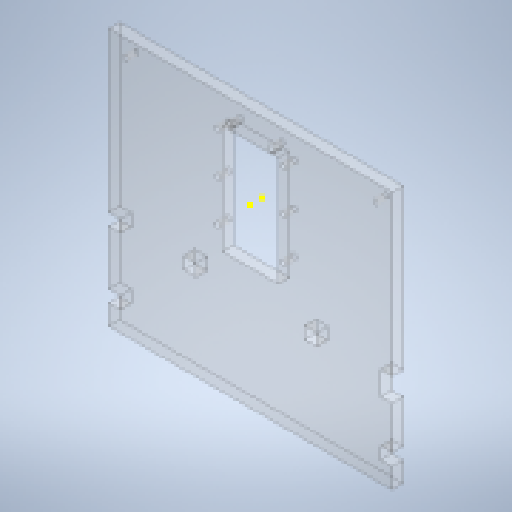
# Autodesk Inventor part: real_waist
Saved by Autodesk Inventor 2024 (Build 280153000, 153)
## iProperties
Created: 2024-09-06
Part Number: real_waist
Material: PMMA 플라스틱
Document SubType Name: Modeling
Designer: Eungang
Density: 1.188 g/cm^3
Appearance: 폴리카보네이트 - 선명
Mass: 126.494 g
Surface Area: 420.568 cm^2
Volume: 106.476 cm^3
Author: Eungang
Autodesk Inventor part; units mm, degrees
ref_plane "YZ Plane" through (0, 0, 0) normal (1, 0, 0) x (0, 1, 0)
ref_plane "XZ Plane" through (0, 0, 0) normal (0, 1, 0) x (-1, 0, 0)
ref_plane "XY Plane" through (0, 0, 0) normal (0, 0, 1) x (1, 0, 0)
sketch "스케치1" plane through (0, 0, 0) normal (0, 0, 1) x (1, 0, 0)
  arc A0 (-19.5808, 6.2636) -> (-20.1, 4.5766) centre (-17.1, 4.5766) ccw projected
  line L0 (-20.1, -39.6766) -> (-20.1, 4.5766) projected
  arc A1 (-20.1, -39.6766) -> (-19.5808, -41.3636) centre (-17.1, -39.6766) ccw projected
  line L1 (-15.8929, -46.7869) -> (-19.5808, -41.3636) projected
  arc A2 (-15.8929, -46.7869) -> (-13.4121, -48.1) centre (-13.4121, -45.1) ccw projected
  line L2 (13.4121, -48.1) -> (-13.4121, -48.1) projected
  arc A3 (13.4121, -48.1) -> (15.8929, -46.7869) centre (13.4121, -45.1) ccw projected
  line L3 (19.5808, -41.3636) -> (15.8929, -46.7869) projected
  arc A4 (19.5808, -41.3636) -> (20.1, -39.6766) centre (17.1, -39.6766) ccw projected
  line L4 (20.1, 4.5766) -> (20.1, -39.6766) projected
  arc A5 (20.1, 4.5766) -> (19.5808, 6.2636) centre (17.1, 4.5766) ccw projected
  line L5 (15.5953, 12.1246) -> (19.5808, 6.2636) projected
  arc A6 (15.5953, 12.1246) -> (13.9414, 13) centre (13.9414, 11) ccw projected
  line L6 (7.65, 13) -> (13.9414, 13) projected
  arc A7 (9.15, 11.5) -> (7.65, 13) centre (7.65, 11.5) ccw projected
  line L7 (9.15, 11.5) -> (9.15, 10) projected
  arc A8 (9.15, 10) -> (11.5, 7.65) centre (11.5, 10) ccw projected
  line L8 (11.5, 7.65) -> (13.5, 7.65) projected
  arc A9 (14.5, 6.65) -> (13.5, 7.65) centre (13.5, 6.65) ccw projected
  line L9 (14.5, 6.65) -> (14.5, -36.15) projected
  arc A10 (13.5, -37.15) -> (14.5, -36.15) centre (13.5, -36.15) ccw projected
  line L10 (13.5, -37.15) -> (11.5, -37.15) projected
  arc A11 (11.5, -37.15) -> (9.15, -39.5) centre (11.5, -39.5) ccw projected
  line L11 (9.15, -39.5) -> (9.15, -41.5) projected
  arc A12 (8.15, -42.5) -> (9.15, -41.5) centre (8.15, -41.5) ccw projected
  line L12 (8.15, -42.5) -> (-8.15, -42.5) projected
  arc A13 (-9.15, -41.5) -> (-8.15, -42.5) centre (-8.15, -41.5) ccw projected
  line L13 (-9.15, -41.5) -> (-9.15, -39.5) projected
  arc A14 (-9.15, -39.5) -> (-11.5, -37.15) centre (-11.5, -39.5) ccw projected
  line L14 (-11.5, -37.15) -> (-13.5, -37.15) projected
  arc A15 (-14.5, -36.15) -> (-13.5, -37.15) centre (-13.5, -36.15) ccw projected
  line L15 (-14.5, -36.15) -> (-14.5, 6.65) projected
  arc A16 (-13.5, 7.65) -> (-14.5, 6.65) centre (-13.5, 6.65) ccw projected
  line L16 (-13.5, 7.65) -> (-11.5, 7.65) projected
  arc A17 (-11.5, 7.65) -> (-9.15, 10) centre (-11.5, 10) ccw projected
  line L17 (-9.15, 10) -> (-9.15, 11.5) projected
  arc A18 (-7.65, 13) -> (-9.15, 11.5) centre (-7.65, 11.5) ccw projected
  line L18 (-13.9414, 13) -> (-7.65, 13) projected
  arc A19 (-13.9414, 13) -> (-15.5953, 12.1246) centre (-13.9414, 11) ccw projected
  line L19 (-19.5808, 6.2636) -> (-15.5953, 12.1246) projected
  circle A20 centre (11, -45.3) radius 1.35 projected
  circle A21 centre (-11, -45.3) radius 1.35 projected
  circle A22 centre (17.3, -40) radius 1.35 projected
  circle A23 centre (-17.3, -40) radius 1.35 projected
  line L20 (-17.3, -18) -> (-17.3, -40)
  line L21 (-17.3, -29) -> (-18.1, -29)
  line L22 (-17.3, -29) -> (-14.5, -29)
  line L23 (-14.5, 6.65) -> (-14.5, -36.15)
  line L24 (-20.1, -27) -> (-20.1, 4.5766)
  line L25 (0, 0) -> (0, -14)
  line L26 (-14.5, 6.65) -> (-14.7, 6.65)
  line L27 (-14.7, 6.65) -> (-14.7, -36.15)
  line L28 (-14.7, -36.15) -> (-14.5, -36.15)
  line L29 (-14.5, 6.65) -> (-18.1, 6.65)
  line L30 (-20.1, 4.65) -> (-20.1, 4.5766)
  arc A24 (-18.1, 6.65) -> (-20.1, 4.65) centre (-18.1, 4.65) ccw
  arc A25 (-20.1, -27) -> (-18.1, -29) centre (-18.1, -27) ccw
  line L31 (20.1, -39.6766) -> (20.1, 4.5766)
  line L32 (17.3, -29) -> (14.5, -29)
  line L33 (14.7, 6.65) -> (14.7, -36.15)
  arc A26 (20.1, 4.65) -> (18.1, 6.65) centre (18.1, 4.65) ccw
  arc A27 (18.1, -29) -> (20.1, -27) centre (18.1, -27) ccw
  line L34 (17.3, -29) -> (18.1, -29)
  line L35 (14.7, 6.65) -> (18.1, 6.65)
  line L36 (-20.1, 6.65) -> (-38.1, 6.65)
  line L37 (-38.1, 6.65) -> (-38.1, -29)
  line L38 (-38.1, -29) -> (-20.1, -29)
  line L39 (-20.1, -29) -> (-20.1, 6.65)
  line L40 (20.1, 6.65) -> (38.1, 6.65)
  line L41 (38.1, 6.65) -> (38.1, -29)
  line L42 (38.1, -29) -> (20.1, -29)
  line L43 (20.1, -29) -> (20.1, 6.65)
  line L44 (-18.1, 6.65) -> (-20.1, 6.65)
  line L45 (-17.3, -29) -> (-20.1, -29)
  line L46 (20.1, -29) -> (18.1, -29)
  line L47 (20.1, 6.65) -> (14.5, 6.65)
  line L48 (-32.5405, -23.1017) -> (-32.4592, -49.1016) projected
  line L49 (-32.5221, -29) -> (-38.1, -29)
  line L50 (-38.1, -29) -> (-38.1, 6.65)
  line L51 (-38.1, 6.65) -> (-32.5221, 6.65)
  line L52 (-32.5221, 6.65) -> (-32.5221, -29)
  line L53 (-32.5221, -29) -> (-32.3221, -29)
  line L54 (-32.3221, -29) -> (-32.3221, 6.65)
  line L55 (32.3221, -29) -> (32.3221, 6.65)
  line L56 (31.5, -1) -> (31.5, -27) projected
  line L57 (-31.5, -1) -> (-31.5, -27) projected
  line L58 (31.5, -29) -> (20.1, -29)
  line L59 (20.1, -29) -> (20.1, 6.65)
  line L60 (20.1, 6.65) -> (31.5, 6.65)
  line L61 (-31.5, -29) -> (-20.1, -29)
  line L62 (-20.1, -29) -> (-20.1, 6.65)
  line L63 (-20.1, 6.65) -> (-31.5, 6.65)
  line L64 (31.5, -29) -> (31.4, -29)
  line L65 (31.4, -29) -> (31.4, -28)
  line L66 (31.4, -28) -> (31.5, -28)
  line L67 (31.5, -28) -> (31.5, -29)
  line L68 (31.4, -28) -> (31.4, 6.65)
  line L69 (-31.5, -29) -> (-31.4, -29)
  line L70 (-31.4, -29) -> (-31.4, 6.65)
  line L71 (31.5, -28) -> (31.5, -27)
  line L72 (-75, -22.9383) -> (-75, -5.0617)
  line L73 (-31.4, -29) -> (-74.8, -29)
  line L74 (-74.8, -29) -> (-74.8, 6.65)
  line L75 (-74.8, 6.65) -> (-31.4, 6.65)
  line L76 (-31.4, 6.65) -> (-31.4, -29)
  line L77 (20.1, 6.65) -> (38.1, 6.65)
  line L78 (38.1, 6.65) -> (38.1, -29)
  line L79 (38.1, -29) -> (20.1, -29)
  line L80 (32.5405, -23.1017) -> (32.4592, -49.1016)
  line L81 (32.5221, -29) -> (38.1, -29)
  line L82 (38.1, -29) -> (38.1, 6.65)
  line L83 (38.1, 6.65) -> (32.5221, 6.65)
  line L84 (32.5221, 6.65) -> (32.5221, -29)
  line L85 (32.5221, -29) -> (32.3221, -29)
  line L86 (32.3221, -29) -> (32.3221, 6.65)
  line L87 (31.5, -1) -> (31.5, -27)
  line L88 (31.5, -29) -> (20.1, -29)
  line L89 (20.1, 6.65) -> (31.5, 6.65)
  line L90 (31.5, -29) -> (31.4, -29)
  line L91 (31.4, -29) -> (31.4, 6.65)
  line L92 (75, -22.9383) -> (75, -5.0617)
  line L93 (31.4, -29) -> (74.8, -29)
  line L94 (74.8, -29) -> (74.8, 6.65)
  line L95 (74.8, 6.65) -> (31.4, 6.65)
  line L96 (31.4, 6.65) -> (31.4, -29)
  circle A28 centre (17.3, 4) radius 1.45
  circle A29 centre (17.3, -18) radius 1.45
  circle A30 centre (-17.3, 4) radius 1.45
  circle A31 centre (-17.3, -18) radius 1.45
  point P0 (-20.1, -29)
  point P1 (-14.7, -29)
  point P2 (-20.0735, 4.9745)
  point P3 (20.0735, 4.9745)
  point P4 (14.7, -29)
  point P5 (-75, -5.0617)
  dimension "d0" = 0.2
  dimension "d1" = 2
  dimension "d4" = 18
  dimension "d5" = 18
  dimension "d16" = 0.2
  dimension "d17" = 0.1
  dimension "d18" = 0.1
  constraints: 148 end point, 27 symmetric about line, 23 point on line, 16 parallel, 12 perpendicular, 11 horizontal, 8 centre point, 8 point on circle, 8 tangent, 6 collinear, 2 vertical, 1 equal radius, 1 midpoint, 6 other
  measures "d0" distance of L15.end L26.end
  measures "d1" radius of A24
  measures "d4" distance of L38.end L37.end
  measures "d5" distance of L41.end L42.end
  measures "d16" distance of L49.start L53.end
  measures "d17" distance of L65.end L66.end
  measures "d18" distance of L61.start L69.end
extrude "돌출1" add sketch "스케치1" along normal blind 6 contours A0 A24 L29 L27 L22 L21 A25 L0 | L39 L44 L19 A0 | A0 L0 L38 L70 L36 L39 | A0 L19 L44 A24 | A25 L45 L0 | L70 L38 L54 L36 | L54 L38 L52 L36 | L52 L38 L37 L36 | L37 L73 L74 L75 | L46 A27 L4 | L4 A5 L43 L40 L68 L65 L42 | A27 L34 L32 L33 L35 A26 A5 L4 | L65 L66 L67 L42 | L67 L66 L68 L40 L55 L42 | A5 L5 L47 L43 | L55 L40 L84 L42 | A26 L47 L5 A5 | L84 L40 L41 L42 | L41 L95 L94 L93
sketch "스케치5" plane through (0, 0, 6) normal (0, 0, 1) x (1, 0, 0)
  arc A0 (19.5808, -20.2636) -> (20.1, -18.5766) centre (17.1, -18.5766) ccw projected
  line L0 (20.1, 25.6766) -> (20.1, -18.5766) projected
  arc A1 (20.1, 25.6766) -> (19.5808, 27.3636) centre (17.1, 25.6766) ccw
  line L1 (15.8929, 32.7869) -> (19.5808, 27.3636) projected
  arc A2 (15.8929, 32.7869) -> (13.4121, 34.1) centre (13.4121, 31.1) ccw projected
  line L2 (-13.4121, 34.1) -> (13.4121, 34.1) projected
  arc A3 (-13.4121, 34.1) -> (-15.8929, 32.7869) centre (-13.4121, 31.1) ccw projected
  line L3 (-19.5808, 27.3636) -> (-15.8929, 32.7869) projected
  arc A4 (-19.5808, 27.3636) -> (-20.1, 25.6766) centre (-17.1, 25.6766) ccw projected
  line L4 (-20.1, -18.5766) -> (-20.1, 25.6766) projected
  arc A5 (-20.1, -18.5766) -> (-19.5808, -20.2636) centre (-17.1, -18.5766) ccw projected
  line L5 (-15.5953, -26.1246) -> (-19.5808, -20.2636) projected
  arc A6 (-15.5953, -26.1246) -> (-13.9414, -27) centre (-13.9414, -25) ccw projected
  line L6 (-7.65, -27) -> (-13.9414, -27) projected
  arc A7 (-9.15, -25.5) -> (-7.65, -27) centre (-7.65, -25.5) ccw projected
  line L7 (-9.15, -25.5) -> (-9.15, -24) projected
  arc A8 (-9.15, -24) -> (-11.5, -21.65) centre (-11.5, -24) ccw projected
  line L8 (-11.5, -21.65) -> (-13.5, -21.65) projected
  arc A9 (-14.5, -20.65) -> (-13.5, -21.65) centre (-13.5, -20.65) ccw projected
  line L9 (-14.5, -20.65) -> (-14.5, 22.15) projected
  arc A10 (-13.5, 23.15) -> (-14.5, 22.15) centre (-13.5, 22.15) ccw projected
  line L10 (-13.5, 23.15) -> (-11.5, 23.15) projected
  arc A11 (-11.5, 23.15) -> (-9.15, 25.5) centre (-11.5, 25.5) ccw projected
  line L11 (-9.15, 25.5) -> (-9.15, 27.5) projected
  arc A12 (-8.15, 28.5) -> (-9.15, 27.5) centre (-8.15, 27.5) ccw projected
  line L12 (-8.15, 28.5) -> (8.15, 28.5) projected
  arc A13 (9.15, 27.5) -> (8.15, 28.5) centre (8.15, 27.5) ccw projected
  line L13 (9.15, 27.5) -> (9.15, 25.5) projected
  arc A14 (9.15, 25.5) -> (11.5, 23.15) centre (11.5, 25.5) ccw projected
  line L14 (11.5, 23.15) -> (13.5, 23.15) projected
  arc A15 (14.5, 22.15) -> (13.5, 23.15) centre (13.5, 22.15) ccw projected
  line L15 (14.5, 22.15) -> (14.5, -20.65) projected
  arc A16 (13.5, -21.65) -> (14.5, -20.65) centre (13.5, -20.65) ccw projected
  line L16 (13.5, -21.65) -> (11.5, -21.65) projected
  arc A17 (11.5, -21.65) -> (9.15, -24) centre (11.5, -24) ccw projected
  line L17 (9.15, -24) -> (9.15, -25.5) projected
  arc A18 (7.65, -27) -> (9.15, -25.5) centre (7.65, -25.5) ccw projected
  line L18 (13.9414, -27) -> (7.65, -27) projected
  arc A19 (13.9414, -27) -> (15.5953, -26.1246) centre (13.9414, -25) ccw projected
  line L19 (19.5808, -20.2636) -> (15.5953, -26.1246) projected
  circle A20 centre (-17.3, -18) radius 1.35 projected
  circle A21 centre (-17.3, 4) radius 1.35 projected
  circle A22 centre (-11, 31.3) radius 1.35 projected
  circle A23 centre (17.3, -18) radius 1.35 projected
  circle A24 centre (17.3, 4) radius 1.35 projected
  line L20 (14.7, 6.65) -> (14.7, -29) projected
  line L21 (14.7, 6.65) -> (20.7, 6.65)
  line L22 (20.7, 6.65) -> (20.7, 26)
  line L23 (20.7, 26) -> (14.7, 26)
  line L24 (14.7, 26) -> (14.7, 6.65)
  line L25 (20.7, 26) -> (14, 26)
  line L26 (11, 28.5) -> (11, 34.5)
  line L27 (11, 34.5) -> (8.15, 34.5)
  line L28 (20.7, 26) -> (11, 26)
  line L29 (11, 29) -> (11, 34.5)
  line L30 (11, 34.5) -> (20.7, 34.5)
  line L31 (20.7, 31.7) -> (20.7, 26)
  line L32 (8.15, 28.5) -> (8.15, 28.7)
  line L33 (8.15, 28.7) -> (11, 28.7)
  line L34 (11, 28.7) -> (11, 34.5)
  line L35 (11, 34.5) -> (8.15, 34.5)
  line L36 (8.15, 34.5) -> (8.15, 28.7)
  line L37 (11, 34.5) -> (8.15, 34.5)
  line L38 (8.15, 34.5) -> (8.15, 34.7)
  line L39 (8.15, 34.7) -> (11, 34.7)
  line L40 (11, 34.7) -> (11, 34.5)
  line L41 (20.7, 34.5) -> (11, 34.5)
  line L42 (11, 34.5) -> (11, 34.7)
  line L43 (11, 34.7) -> (17.7, 34.7)
  line L44 (20.7, 34.7) -> (20.7, 34.5)
  line L45 (8.15, 34.7) -> (3, 34.7)
  line L46 (0, 31.7) -> (0, 28.7)
  line L47 (0, 28.7) -> (8.15, 28.7)
  line L48 (8.15, 28.7) -> (8.15, 34.7)
  arc A25 (20.7, 31.7) -> (17.7, 34.7) centre (17.7, 31.7) ccw
  arc A26 (11, 29) -> (14, 26) centre (14, 29) ccw
  arc A27 (3, 34.7) -> (0, 31.7) centre (3, 31.7) ccw
  line L49 (0, 0) -> (0, -14)
  arc A28 (-19.5808, 27.3636) -> (-20.1, 25.6766) centre (-17.1, 25.6766) ccw
  line L50 (-15.8929, 32.7869) -> (-19.5808, 27.3636)
  arc A29 (-13.4121, 34.1) -> (-15.8929, 32.7869) centre (-13.4121, 31.1) ccw
  arc A30 (-8.15, 28.5) -> (-9.15, 27.5) centre (-8.15, 27.5) ccw
  line L51 (-9.15, 27.5) -> (-9.15, 25.5)
  arc A31 (-11.5, 23.15) -> (-9.15, 25.5) centre (-11.5, 25.5) ccw
  line L52 (-11.5, 23.15) -> (-13.5, 23.15)
  arc A32 (-13.5, 23.15) -> (-14.5, 22.15) centre (-13.5, 22.15) ccw
  line L53 (-14.7, 6.65) -> (-20.7, 6.65)
  line L54 (-20.7, 6.65) -> (-20.7, 26)
  line L55 (-20.7, 26) -> (-14.7, 26)
  line L56 (-14.7, 26) -> (-14.7, 6.65)
  line L57 (-20.7, 26) -> (-14, 26)
  line L58 (-11, 28.5) -> (-11, 34.5)
  line L59 (-11, 34.5) -> (-8.15, 34.5)
  line L60 (-20.7, 26) -> (-11, 26)
  line L61 (-11, 29) -> (-11, 34.5)
  line L62 (-11, 34.5) -> (-20.7, 34.5)
  line L63 (-20.7, 31.7) -> (-20.7, 26)
  line L64 (-8.15, 28.5) -> (-8.15, 28.7)
  line L65 (-8.15, 28.7) -> (-11, 28.7)
  line L66 (-11, 28.7) -> (-11, 34.5)
  line L67 (-11, 34.5) -> (-8.15, 34.5)
  line L68 (-8.15, 34.5) -> (-8.15, 28.7)
  line L69 (-11, 34.5) -> (-8.15, 34.5)
  line L70 (-8.15, 34.5) -> (-8.15, 34.7)
  line L71 (-8.15, 34.7) -> (-11, 34.7)
  line L72 (-11, 34.7) -> (-11, 34.5)
  line L73 (-20.7, 34.5) -> (-11, 34.5)
  line L74 (-11, 34.5) -> (-11, 34.7)
  line L75 (-11, 34.7) -> (-17.7, 34.7)
  line L76 (-20.7, 34.7) -> (-20.7, 34.5)
  line L77 (-8.15, 34.7) -> (-3, 34.7)
  line L78 (0, 28.7) -> (-8.15, 28.7)
  line L79 (-8.15, 28.7) -> (-8.15, 34.7)
  arc A33 (-17.7, 34.7) -> (-20.7, 31.7) centre (-17.7, 31.7) ccw
  arc A34 (-14, 26) -> (-11, 29) centre (-14, 29) ccw
  arc A35 (0, 31.7) -> (-3, 34.7) centre (-3, 31.7) ccw
  line L80 (3, 34.7) -> (-3, 34.7)
  circle A36 centre (17.3, 26) radius 1.45
  circle A37 centre (11, 31.3) radius 1.45
  circle A38 centre (-17.3, 26) radius 1.45
  circle A39 centre (-11, 31.3) radius 1.45
  line L81 (8.15, 28.5) -> (14.5, 28.5)
  line L82 (14.5, 28.5) -> (14.5, 22.15)
  line L83 (14.5, 22.15) -> (8.15, 22.15)
  line L84 (8.15, 22.15) -> (8.15, 28.5)
  line L85 (-14.5, -20.65) -> (-7.65, -20.65)
  line L86 (-7.65, -20.65) -> (-7.65, -27)
  line L87 (-7.65, -27) -> (-14.5, -27)
  line L88 (-14.5, -27) -> (-14.5, -20.65)
  line L89 (8.15, 22.15) -> (-7.65, 22.15)
  line L90 (-7.65, 22.15) -> (-7.65, -20.65)
  line L91 (-7.65, -20.65) -> (8.15, -20.65)
  line L92 (8.15, -20.65) -> (8.15, 22.15)
  line L93 (11, 28.7) -> (14.5, 28.7)
  line L94 (14.5, 28.7) -> (14.5, 22.15)
  line L95 (14.5, 22.15) -> (11, 22.15)
  line L96 (11, 22.15) -> (11, 28.7)
  line L97 (-11, 28.7) -> (-14.7, 28.7)
  line L98 (-14.7, 28.7) -> (-14.7, 26)
  line L99 (-14.7, 26) -> (-11, 26)
  line L100 (-11, 26) -> (-11, 28.7)
  line L101 (7.65, -27) -> (14.5, -27)
  line L102 (14.5, -27) -> (14.5, -20.65)
  line L103 (14.5, -20.65) -> (7.65, -20.65)
  line L104 (7.65, -20.65) -> (7.65, -27)
  line L105 (14.7, 26) -> (14.5, 26)
  line L106 (14.5, 26) -> (14.5, 28.7)
  line L107 (14.5, 28.7) -> (14.7, 28.7)
  line L108 (14.7, 28.7) -> (14.7, 26)
  point P0 (-17.3, 4)
  point P1 (-11, 29.85)
  point P2 (-11, 29.95)
  point P3 (-11, 32.65)
  point P4 (-11, 32.75)
  point P5 (-11.015, 28.7)
  point P6 (11.015, 28.7)
  dimension "d19" = 6
  dimension "d20" = 6
  dimension "d21" = 0.2
  dimension "d22" = 0.2
  dimension "d23" = 3
  constraints: 176 end point, 34 symmetric about line, 26 parallel, 24 point on circle, 16 centre point, 15 horizontal, 13 perpendicular, 8 tangent, 6 point on line, 2 equal radius, 2 vertical, 10 other
  measures "d19" distance of L23.end L22.end
  measures "d20" distance of L26.end L26.start
  measures "d21" distance of L12.end L32.end
  measures "d22" distance of L37.end L38.end
  measures "d23" radius of A25
extrude "돌출5" add sketch "스케치5" against normal blind 6 contours L21 L24 L23 A36 A1 L0 | L0 A1 L23 L22 L21 | L23 A36 L108 L107 L93 A26 L26 A37 L2 A2 L1 A1 | A1 L1 A2 L2 L26 L30 A25 L31 L23 | L30 L40 L43 A25 | L26 L2 L36 L27 | L27 L38 L39 L40 | L26 A37 L33 L36 L2 | L36 L2 A27 L45 L38 | L47 L46 A27 L2 L36 | L65 L58 A39 L2 L68 | L68 L2 A35 L46 L78 | A27 A35 L2 | L2 A35 L80 A27 | L68 L70 L77 A35 L2 | L2 L58 L59 L68 | A34 L97 L98 L55 A38 A4 L3 A3 L2 L58 A39 | L2 A3 L3 A4 L55 L63 A33 L62 L58 | L59 L72 L71 L70 | L62 A33 L75 L72 | L53 L54 L55 A4 L4 | L4 A4 L55 A38 L56 L53
sketch "스케치15" plane through (0, 0, 0) normal (0, 0, -1) x (-1, 0, 0)
  circle A0 centre (0, -14) radius 1.6 projected
  line L0 (-29, 25.8) -> (29, 25.8) projected
  line L1 (-29, 19.8) -> (-29, 25.8) projected
  line L2 (-35, 19.8) -> (-29, 19.8) projected
  line L3 (-35, 25.8) -> (-35, 19.8) projected
  line L4 (-69, 25.8) -> (-35, 25.8) projected
  line L5 (-69, 19.8) -> (-69, 25.8) projected
  line L6 (-75, 19.8) -> (-69, 19.8) projected
  line L7 (-75, -93.4) -> (-75, 19.8) projected
  line L8 (-69, -93.4) -> (-75, -93.4) projected
  line L9 (-69, -99.4) -> (-69, -93.4) projected
  line L10 (-35, -99.4) -> (-69, -99.4) projected
  line L11 (-35, -93.4) -> (-35, -99.4) projected
  line L12 (-29, -93.4) -> (-35, -93.4) projected
  line L13 (-29, -99.4) -> (-29, -93.4) projected
  line L14 (29, -99.4) -> (-29, -99.4) projected
  line L15 (29, -93.4) -> (29, -99.4) projected
  line L16 (35, -93.4) -> (29, -93.4) projected
  line L17 (35, -99.4) -> (35, -93.4) projected
  line L18 (69, -99.4) -> (35, -99.4) projected
  line L19 (69, -93.4) -> (69, -99.4) projected
  line L20 (75, -93.4) -> (69, -93.4) projected
  line L21 (75, 19.8) -> (75, -93.4) projected
  line L22 (69, 19.8) -> (75, 19.8) projected
  line L23 (69, 25.8) -> (69, 19.8) projected
  line L24 (35, 25.8) -> (69, 25.8) projected
  line L25 (35, 19.8) -> (35, 25.8) projected
  line L26 (29, 19.8) -> (35, 19.8) projected
  line L27 (29, 25.8) -> (29, 19.8) projected
  line L28 (-14.7, -29) -> (-74.8, -29) projected
  line L29 (-74.8, -29) -> (75.2, -29)
  line L30 (75.2, -29) -> (75.2, -99.4)
  line L31 (75.2, -99.4) -> (-74.8, -99.4)
  line L32 (-74.8, -99.4) -> (-74.8, -29)
  line L33 (-69, -76.4) -> (-69, -82.4) projected
  line L34 (-69, -76.4) -> (-75, -76.4) projected
  line L35 (-75, -82.4) -> (-75, -76.4) projected
  line L36 (-69, -82.4) -> (-75, -82.4) projected
  line L37 (-69, -41.4) -> (-75, -41.4) projected
  line L38 (-75, -41.4) -> (-75, -47.4) projected
  line L39 (-69, -47.4) -> (-75, -47.4) projected
  line L40 (-69, -41.4) -> (-69, -47.4) projected
  line L41 (-69, -47.4) -> (-69, -53.4) projected
  line L42 (-69, -47.4) -> (-75, -47.4) projected
  line L43 (-75, -53.4) -> (-75, -47.4) projected
  line L44 (-69, -53.4) -> (-75, -53.4) projected
  line L45 (-29, -41.4) -> (-35, -41.4) projected
  line L46 (-35, -41.4) -> (-35, -47.4) projected
  line L47 (-29, -47.4) -> (-35, -47.4) projected
  line L48 (-29, -41.4) -> (-29, -47.4) projected
  line L49 (75, -76.4) -> (75, -82.4) projected
  line L50 (75, -76.4) -> (69, -76.4) projected
  line L51 (69, -82.4) -> (69, -76.4) projected
  line L52 (75, -82.4) -> (69, -82.4) projected
  line L53 (35, -41.4) -> (35, -47.4) projected
  line L54 (69, -47.4) -> (35, -47.4) projected
  line L55 (69, -41.4) -> (69, -47.4) projected
  line L56 (35, -41.4) -> (69, -41.4) projected
  line L57 (75, -41.4) -> (69, -41.4) projected
  line L58 (69, -41.4) -> (69, -47.4) projected
  line L59 (75, -47.4) -> (69, -47.4) projected
  line L60 (75, -41.4) -> (75, -47.4) projected
  line L61 (35, -41.4) -> (29, -41.4) projected
  line L62 (29, -41.4) -> (29, -47.4) projected
  line L63 (35, -47.4) -> (29, -47.4) projected
  line L64 (35, -41.4) -> (35, -47.4) projected
  point P0 (0, 0)
  point P1 (75, -29)
  point P2 (-74.8, -93.4)
  point P3 (-74.8, -41.4)
  point P4 (-74.8, -47.4)
  point P5 (-74.8, -53.4)
  point P6 (-74.8, -76.4)
  point P7 (-74.8, -82.4)
  constraints: 8 end point, 2 parallel, 1 horizontal, 1 perpendicular, 1 other
extrude "돌출10" add sketch "스케치15" against normal blind 6 contours A0 | L0 L27 L26 L25 L24 L23 L22 L21 L29 L28 L32 L37 L7 L6 L5 L4 L3 L2 L1 | L37 L32 L39 L7 | L29 L30 L31 L19 L20 L21 | L21 L57 L56 L61 L62 L63 L54 L59 L50 L51 L52 L20 L19 L18 L17 L16 L15 L14 L13 L12 L11 L10 L9 L8 L32 L36 L33 L34 L44 L41 L40 L37 L28 L29 | L39 L32 L44 L7 | L21 L59 L55 L57 | L44 L32 L34 L7 | L55 L54 L53 L56 | L34 L32 L36 L7 | L21 L52 L51 L50 | L36 L32 L8 L7 | L31 L15 L16 L17 | L8 L9 L31 L32 | L31 L11 L12 L13
sketch "스케치16" plane through (0, 0, 0) normal (0, 0, -1) x (-1, 0, 0)
  point P0 (0, 0)
feature "두껍게 하기1" [suppressed]
feature "두껍게 하기2" [suppressed]
feature "두껍게 하기3" [suppressed]
feature "두껍게 하기4" [suppressed]
feature "두껍게 하기5" [suppressed]
feature "두껍게 하기6" [suppressed]
feature "두껍게 하기7" [suppressed]
feature "두껍게 하기8" [suppressed]
thicken "두껍게 하기9" operation cut thickness 0.2 both sides no extend neighbours no toward (1, 0, 0) faces at (-29, -45.4, 2) (-31, -41.4, 2) (-33, -47.4, 2) (-35, -43.4, 2)
thicken "두껍게 하기10" operation cut thickness 0.2 both sides no extend neighbours no toward (-1, 0, 0) faces at (29, -43.4, 2) (31, -47.4, 2) (33, -41.4, 2) (35, -45.4, 2)
thicken "두껍게 하기11" operation cut thickness 0.2 both sides no extend neighbours no toward (0, 0, -1) faces at (-9.7333, -82.1333, 6)
sketch "스케치19" plane through (-68.8, -99.4, 0) normal (-1, 0, 0) x (0, 0, 1)
  line L0 (5.8, 6.2) -> (5.8, 0) projected
  line L1 (0, 6.2) -> (5.8, 6.2) projected
  line L2 (5.8, 0) -> (0, 0)
  line L3 (0, 0) -> (0, 6.2)
  line L4 (0, 6.2) -> (5.8, 6.2)
  line L5 (5.8, 6.2) -> (5.8, 0)
  point P0 (0, 99.4)
  constraints: 8 end point, 2 parallel, 1 horizontal, 1 perpendicular
extrude "돌출13" [suppressed]
sketch "스케치20" plane through (-75, -93.4, 5.8) normal (0, 0, 1) x (1, 0, 0)
  line L0 (150, 113.2) -> (150, 0) projected
  arc A0 (95.7, 125.1) -> (92.7, 128.1) centre (92.7, 125.1) ccw projected
  line L1 (150, 99.85) -> (92.7, 99.85)
  line L2 (92.7, 99.85) -> (92.7, 128.1)
  line L3 (92.7, 128.1) -> (150, 128.1)
  line L4 (150, 128.1) -> (150, 99.85)
  arc A1 (57.3, 128.1) -> (54.3, 125.1) centre (57.3, 125.1) ccw projected
  line L5 (57.3, 128.1) -> (0, 128.1)
  line L6 (0, 128.1) -> (0, 99.85)
  line L7 (0, 99.85) -> (57.3, 99.85)
  line L8 (57.3, 99.85) -> (57.3, 128.1)
  point P0 (75, 93.4)
  point P1 (150, 52)
  constraints: 16 end point, 4 parallel, 2 horizontal, 2 perpendicular, 1 point on line
extrude "돌출14" add sketch "스케치20" against normal blind 5.8
sketch "스케치21" plane through (-75, 34.7, 5.8) normal (0, 0, 1) x (1, 0, 0)
  point P0 (75, -34.7)
sketch "스케치22" plane through (-75, 34.7, 0) normal (0, 1, 0) x (1, 0, 0)
  line L0 (150, 0) -> (149.8, 0) projected
  line L1 (150, -5.8) -> (149.8, -5.8) projected
  line L2 (150, 0) -> (0, 0)
  line L3 (0, 0) -> (0, -5.8)
  line L4 (0, -5.8) -> (150, -5.8)
  line L5 (150, -5.8) -> (150, 0)
  line L6 (150, -5.8) -> (0, -5.8)
  line L7 (0, -5.8) -> (0, 0.2)
  line L8 (0, 0.2) -> (150, 0.2)
  line L9 (150, 0.2) -> (150, -5.8)
  point P0 (75, 0)
  point P1 (0, 0)
  point P2 (150, 0)
  dimension "d109" = 6
  constraints: 16 end point, 4 parallel, 2 horizontal, 2 perpendicular
  measures "d109" distance of L6.end L7.end
extrude "돌출15" add sketch "스케치22" against normal blind 127.9
sketch "스케치23" plane through (75, 34.7, -0.2) normal (0, 0, -1) x (-1, 0, 0)
  line L0 (0, -128.1) -> (0, 0) projected
  line L1 (0, 0) -> (150, 0) projected
  line L2 (150, -127.9) -> (150, -117.3) projected
  line L3 (150, -117.3) -> (150, -75.9)
  line L4 (150, 0) -> (150, -127.9) projected
  line L5 (0, -117.3) -> (0, -75.9)
  line L6 (0, 0) -> (150, 0) projected
  line L7 (0, 0) -> (0, -127.9) projected
  line L8 (150, -127.9) -> (0, -127.9) projected
  line L9 (150, 0) -> (150, -127.9) projected
  circle A0 centre (57.7, -8.7) radius 1.45
  circle A1 centre (92.3, -8.7) radius 1.45
  line L10 (0.2, -134.1) -> (150.2, -134.1) projected
  line L11 (150, -63.7) -> (150, 0) projected
  line L12 (150.2, -63.7) -> (150, -63.7) projected
  line L13 (150.2, -134.1) -> (150.2, -63.7) projected
  line L14 (0.2, -128.1) -> (0.2, -134.1) projected
  line L15 (0, -128.1) -> (0.2, -128.1) projected
  point P0 (75, -34.7)
  point P1 (57.3, -10.0937)
  point P2 (92.7, -10.0937)
  point P3 (150, -82.3)
  point P4 (150, -110.9)
  constraints: 4 end point, 1 collinear, 6 other
extrude "돌출16" cut sketch "스케치23" against normal blind 6 contours A0 | A1
sketch "스케치24" plane through (-75, 34.7, 5.8) normal (0, 1, 0) x (1, 0, 0)
  line L0 (150, 0) -> (0, 0) projected
  line L1 (150, 0) -> (150, 6) projected
  line L2 (150, 6) -> (0, 6) projected
  line L3 (0, 0) -> (0, 6) projected
  point P0 (75, 5.8)
extrude "돌출17" add sketch "스케치24" along normal blind 8
thicken "두껍게 하기13" operation cut thickness 0.2 both sides no extend neighbours no toward (0, 0, 1) faces at (-5.7084, -53.9465, -0.2)
thicken "두껍게 하기14" operation add thickness 0.364 both sides no extend neighbours no toward (0, 1, 0) faces at (25, 42.7, 1.9333)
sketch "스케치25" plane through (-75, -93.2, 5.8) normal (0, 0, 1) x (1, 0, 0)
  point P0 (75, 93.2)
feature "두껍게 하기15" [suppressed]
sketch "스케치29" plane through (-75, -93.2, 5.8) normal (0, 0, 1) x (1, 0, 0)
  circle A0 centre (9.2, 133.2636) radius 1.35 projected
  circle A1 centre (141, 133.2636) radius 1.35 projected
  circle A2 centre (140.8, 55) radius 1.35 projected
  circle A3 centre (9.2, 55) radius 1.35 projected
  point P0 (75, 93.2)
extrude "돌출21" cut sketch "스케치29" against normal up to next contours A0 | A2 | A3
sketch "스케치30" plane through (-75, -93.2, 5.8) normal (0, 0, 1) x (1, 0, 0)
  circle A0 centre (9.2, 55) radius 1.35 projected
  line L0 (6.2, 52) -> (6.2, 64) projected
  line L1 (12.2, 52) -> (6.2, 52) projected
  line L2 (12.2, 64) -> (12.2, 52) projected
  line L3 (6.2, 64) -> (12.2, 64) projected
  circle A1 centre (9.2, 133.2636) radius 1.35 projected
  line L4 (6.2, 136.2636) -> (6.2, 124.2636) projected
  line L5 (6.2, 124.2636) -> (12.2, 124.2636) projected
  line L6 (12.2, 124.2636) -> (12.2, 136.2636) projected
  line L7 (12.2, 136.2636) -> (6.2, 136.2636) projected
  point P0 (75, 93.2)
sketch "스케치31" plane through (-75, -99.4, 5.8) normal (0, 0, 1) x (1, 0, 0)
  line L0 (-6, -0.1644) -> (156, -0.1644) projected
  line L1 (156, -0.1644) -> (156, 5.8356) projected
  line L2 (-6, 5.8356) -> (156, 5.8356) projected
  line L3 (-6, -0.1644) -> (-6, 5.8356) projected
  line L4 (4.32, 31.1) -> (9.22, 31.1) projected
  line L5 (0, 142.4636) -> (-6, 142.4636) projected
  line L6 (-6, 142.4636) -> (-6, 5.8356) projected
  line L7 (0, 5.8356) -> (-6, 5.8356) projected
  line L8 (0, 142.4636) -> (0, 5.8356) projected
  point P0 (75, 99.4)
sketch "스케치32" plane through (-75, -99.4, 5.8) normal (0, 0, 1) x (1, 0, 0)
  line L0 (0, 142.4636) -> (-6, 142.4636) projected
  line L1 (-6, 142.4636) -> (-6, 5.8356) projected
  line L2 (0, 5.8356) -> (-6, 5.8356) projected
  line L3 (0, 142.4636) -> (0, 5.8356) projected
  line L4 (149.8, 0) -> (-0.2, 0) projected
  line L5 (150, 119.2) -> (150, 6) projected
  line L6 (0, 0) -> (150, 0)
  line L7 (150, 0) -> (150, 6)
  line L8 (150, 6) -> (0, 6)
  line L9 (0, 6) -> (0, 0)
  point P0 (75, 99.4)
  point P1 (150, 0)
  point P2 (150, 45.8)
  point P3 (0, 6)
  dimension "d132" = 6
  constraints: 9 end point, 2 parallel, 1 horizontal, 1 perpendicular
  measures "d132" distance of L5.end L6.end
extrude "돌출22" cut sketch "스케치32" against normal blind 6 contours L8 L7 L6 L4 L9 L3
feature "두껍게 하기16" [suppressed]
feature "두껍게 하기17" [suppressed]
feature "두껍게 하기19" [suppressed]
sketch "스케치34" plane through (68.8, -53.6, 5.8) normal (0, 0, 1) x (1, 0, 0)
  circle A0 centre (-3, 93.6636) radius 1.35 projected
  point P0 (-68.8, 53.6)
extrude "돌출24" cut sketch "스케치34" against normal up to next
thicken "두껍게 하기20" operation cut thickness 0.2 both sides no extend neighbours no toward (-1, 0, 0) faces at (75, 40.276, 3.8667) (75, -50.7, 3.8667)
thicken "두껍게 하기21" operation cut thickness 0.2 both sides no extend neighbours no toward (1, 0, 0) faces at (-75, -4.9787, 3.8667)
thicken "두껍게 하기22" operation cut thickness 0.4 both sides no extend neighbours no toward (1, 0, 0) faces at (-75.2, -75.9333, 1.9333)
thicken "두껍게 하기23" operation cut thickness 0.036 both sides no extend neighbours no toward (0, 1, 0) faces at (24.9333, -93.4, 3.8667)
